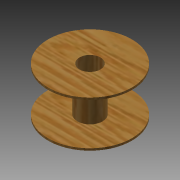
# Autodesk Inventor part: roll
Saved by Autodesk Inventor 2013 (Build 170138000, 138)
## iProperties
Created: 2014-10-20
Part Number: roll
Material: Plywood, Finish
Document SubType Name: Modeling
Designer: Masta
Density: 0.552 g/cm^3
Mass: 81.2887 g
Surface Area: 628.319 cm^2
Volume: 147.262 cm^3
Author: Masta
Autodesk Inventor part; units mm, degrees
ref_plane "YZ Plane" through (0, 0, 0) normal (1, 0, 0) x (0, 1, 0)
ref_plane "XZ Plane" through (0, 0, 0) normal (0, 1, 0) x (-1, 0, 0)
ref_plane "XY Plane" through (0, 0, 0) normal (0, 0, 1) x (1, 0, 0)
sketch "Sketch1" plane through (0, 0, 0) normal (0, 0, 1) x (1, 0, 0)
  circle A0 centre (0, 0) radius 25
  circle A1 centre (0, 0) radius 100
  circle A2 centre (0, 0) radius 30
  dimension "d0" = 50
  dimension "d1" = 200
  dimension "d2" = 5
  constraints: 3 centre point, 3 coincident
  measures "d0" diameter of A0
  measures "d1" diameter of A1
  measures "d2" radial gap between concentric circles of A0 A2
extrude "Extrusion1" add sketch "Sketch1" along normal blind 5 contours A1 | A2
move or copy body "Move Body1" bodies to move or copy 1 copy no translate (0, 0, 50)
mirror "Mirror1" about plane through (0, 0, 0) normal (0, 0, 1)
extrude "Extrusion2" add sketch "Sketch1" against normal up to surface (110 mm away) from surface at 55 contours A2
body "Solid1"
